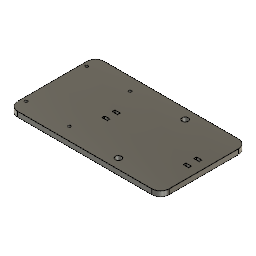
assembly v3 (Autodesk Fusion 360 archive; units mm, degrees)
design "base_assem"
Autodesk Fusion 360 part; units mm, degrees
sketch "Sketch1" plane through (0, 0, 0) normal (0, 0, 1) x (1, 0, 0)
  line L0 (10, 0) -> (165, 0)
  line L1 (175, 10) -> (175, 90)
  line L2 (165, 100) -> (10, 100)
  line L3 (0, 90) -> (0, 10)
  line L4 (5, 85) -> (55, 85)
  line L5 (55, 85) -> (55, 15)
  line L6 (55, 15) -> (5, 15)
  line L7 (5, 15) -> (5, 85)
  line L8 (5, 50) -> (0, 50)
  circle A0 centre (5, 85) radius 1.5
  circle A1 centre (55, 85) radius 1.5
  circle A2 centre (5, 15) radius 1.5
  circle A3 centre (55, 15) radius 1.5
  line L9 (55, 100) -> (55, 0)
  line L10 (65, 100) -> (65, 0)
  line L11 (165, 0) -> (165, 100)
  line L12 (65, 57.5) -> (71, 57.5)
  line L13 (71, 57.5) -> (71, 42.5)
  line L14 (71, 42.5) -> (65, 42.5)
  line L15 (65, 42.5) -> (65, 57.5)
  line L16 (65, 57.5) -> (71, 57.5)
  line L17 (71, 57.5) -> (71, 54.5)
  line L18 (71, 54.5) -> (65, 54.5)
  line L19 (65, 54.5) -> (65, 57.5)
  line L20 (71, 42.5) -> (65, 42.5)
  line L21 (65, 42.5) -> (65, 45.5)
  line L22 (65, 45.5) -> (71, 45.5)
  line L23 (71, 45.5) -> (71, 42.5)
  line L24 (65, 100) -> (165, 100)
  line L25 (115, 100) -> (115, 0)
  line L26 (159, 57.5) -> (159, 42.5)
  line L27 (159, 54.5) -> (165, 54.5)
  line L28 (165, 57.5) -> (159, 57.5)
  line L29 (165, 45.5) -> (159, 45.5)
  line L30 (159, 42.5) -> (165, 42.5)
  circle A4 centre (115, 88.5) radius 3.5
  circle A5 centre (115, 11.5) radius 3.5
  line L31 (115, 88.5) -> (115, 11.5)
  arc A6 (10, 100) -> (0, 90) centre (10, 90) ccw
  arc A7 (0, 10) -> (10, 0) centre (10, 10) ccw
  arc A8 (175, 90) -> (165, 100) centre (165, 90) ccw
  arc A9 (165, 0) -> (175, 10) centre (165, 10) ccw
  point P0 (0, 100)
  point P1 (65, 50)
  point P2 (65, 50)
  point P3 (115, 50)
  point P4 (115, 50)
  dimension "d1" = 50
  dimension "d2" = 70
  dimension "d3" = 100
  dimension "d4" = 90
  dimension "d5" = 5
  dimension "d6" = 3
  dimension "d7" = 3
  dimension "d8" = 3
  dimension "d9" = 3
  dimension "d11" = 120
  dimension "d12" = 10
  dimension "d13" = 10
  dimension "d14" = 6
  dimension "d15" = 15
  dimension "d16" = 3
  dimension "d17" = 3
  dimension "d18" = 77
  dimension "d19" = 7
  dimension "d20" = 7
  dimension "d21" = 10
  dimension "d22" = 10
  dimension "d23" = 10
  dimension "d24" = 10
  constraint horizontal L0
  constraint vertical L1
  constraint horizontal L2
  constraint vertical L3
  constraint horizontal L4
  constraint vertical L5
  constraint horizontal L6
  constraint vertical L7
  constraint midpoint L7 L8.start
  constraint coincident L4.start L7.end
  constraint coincident L4.end L5.start
  constraint coincident L6.end L7.start
  constraint coincident L5.end L6.start
  constraint coincident L0 L9.end
  constraint perpendicular L0 L9
  constraint coincident L2 L10.start
  constraint coincident L0 L10.end
  constraint perpendicular L0 L10
  constraint coincident L0 L11.start
  constraint coincident L2 L11.end
  constraint perpendicular L2 L11
  constraint coincident L4.end L9
  constraint horizontal L12
  constraint vertical L13
  constraint horizontal L14
  constraint vertical L15
  constraint horizontal L16
  constraint vertical L17
  constraint horizontal L18
  constraint vertical L19
  constraint coincident L13 L17.end
  constraint horizontal L20
  constraint vertical L21
  constraint horizontal L22
  constraint vertical L23
  constraint coincident L15 L21.end
  constraint midpoint L10 P2
  constraint midpoint L15 P2
  constraint coincident P2 P1
  constraint midpoint L24 L25.start
  constraint coincident L0 L25.end
  constraint perpendicular L0 L25
  constraint symmetric L12.start L25 L28.start
  constraint symmetric L12.end L25 L26.start
  constraint symmetric L13.end L25 L26.end
  constraint symmetric L17.end L25 L27.start
  constraint symmetric L18.end L25 L27.end
  constraint symmetric L14.end L25 L30.end
  constraint symmetric L21.end L25 L29.start
  constraint symmetric L22.end L25 L29.end
  constraint coincident L25 A4.centre
  constraint coincident L25 A5.centre
  constraint coincident A4.centre L31.start
  constraint coincident A5.centre L31.end
  constraint midpoint L31 P4
  constraint midpoint L25 P4
  constraint coincident P4 P3
  constraint coincident L3 L8.end
  constraint coincident P0 L2
  constraint coincident P0 L3
  constraint tangent L2 A6
  constraint tangent L3 A6
  constraint coincident origin L0
  constraint coincident origin L3
  constraint tangent L0 A7
  constraint tangent L3 A7
  constraint tangent L1 A8
  constraint tangent L2 A8
  constraint tangent L0 A9
  constraint tangent L1 A9
  measures "d1" distance of L4.start L4.end
  measures "d2" distance of L4.start L6.end
  measures "d3" distance of origin P0
  measures "d4" angle of L3 L8
  measures "d5" distance of L8.start L8.end
  measures "d6" diameter of A0
  measures "d7" diameter of A1
  measures "d8" diameter of A3
  measures "d9" diameter of A2
  measures "d11" distance of L1 L9
  measures "d12" distance of L9 L10
  measures "d13" distance of L1 L11
  measures "d14" distance of L12.start L12.end
  measures "d15" distance of L12.end L13.end
  measures "d16" distance of L16 L18
  measures "d17" distance of L14 L22
  measures "d18" distance of A4.centre A5.centre
  measures "d19" diameter of A4
  measures "d20" diameter of A5
  measures "d21" radius of A6
  measures "d22" radius of A7
  measures "d23" radius of A8
  measures "d24" radius of A9
extrude "Extrude1" add sketch "Sketch1" along normal blind 6 contours L0 L3 L6 L7 L8 A2 A3 L9 A7 | L0 L2 L5 A1 A3 L9 L10 L15 L19 L21 | L0 L2 L10 L12 L13 L14 L16 L17 L20 L23 L24 L25 A4 A5 L31 | L2 L3 L4 L7 L8 A0 A1 L9 A6 | L0 L2 L11 L24 L25 L26 L28 L30 A4 A5 L31 | L4 L5 L6 L7 A0 A1 A2 A3 L9 | L1 L11 A8 A9 | L10 L13 L15 L18 L22 | L11 L26 L27 L29
equation "d18 = ( ( 70 + 84 ) / 2 ) * 1 mm"

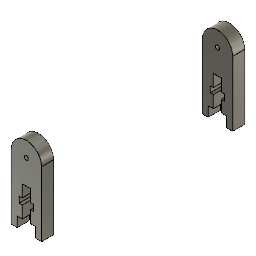
design "rotor_mount_assem"
Autodesk Fusion 360 part; units mm, degrees
sketch "Sketch1" plane through (0, 0, 0) normal (0, 1, 0) x (1, 0, 0)
  circle A0 centre (0, 0) radius 28.5
  line L0 (-9, 27.0416) -> (9, 27.0416)
  line L1 (-27.3663, -7.9584) -> (-39.2742, -7.9584)
  line L2 (-49.2742, 2.0416) -> (-49.2742, 27.0416)
  line L3 (-49.2742, 27.0416) -> (-9, 27.0416)
  line L4 (-41.2742, 27.0416) -> (-34.2742, 27.0416)
  line L5 (-34.2742, 27.0416) -> (-34.2742, 2.0416)
  line L6 (-34.2742, 2.0416) -> (-41.2742, 2.0416)
  line L7 (-41.2742, 2.0416) -> (-41.2742, 27.0416)
  line L8 (-41.2742, 2.0416) -> (-49.2742, 2.0416)
  line L9 (-49.2742, 2.0416) -> (-34.2742, 2.0416)
  line L10 (-28.4268, 2.0416) -> (-34.2742, 2.0416)
  line L11 (-44.2742, 11.0416) -> (-31.2742, 11.0416)
  line L12 (-31.2742, 11.0416) -> (-31.2742, 18.0416)
  line L13 (-31.2742, 18.0416) -> (-44.2742, 18.0416)
  line L14 (-44.2742, 18.0416) -> (-44.2742, 11.0416)
  line L15 (-37.7742, 18.0416) -> (-37.7742, 27.0416)
  line L16 (-44.2742, 14.5416) -> (-41.2742, 14.5416)
  line L17 (-44.2742, 11.0416) -> (-49.2742, 11.0416)
  line L18 (-31.2742, 11.0416) -> (-26.2742, 11.0416)
  arc A1 (-49.2742, 2.0416) -> (-39.2742, -7.9584) centre (-39.2742, 2.0416) ccw
  line L19 (0, 27.0416) -> (0, 0)
  line L20 (27.3663, -7.9584) -> (39.2742, -7.9584)
  arc A2 (39.2742, -7.9584) -> (49.2742, 2.0416) centre (39.2742, 2.0416) ccw
  line L21 (49.2742, 2.0416) -> (49.2742, 27.0416)
  line L22 (49.2742, 27.0416) -> (9, 27.0416)
  line L23 (31.2742, 18.0416) -> (44.2742, 18.0416)
  line L24 (31.2742, 11.0416) -> (31.2742, 18.0416)
  line L25 (44.2742, 11.0416) -> (31.2742, 11.0416)
  line L26 (44.2742, 18.0416) -> (44.2742, 11.0416)
  line L27 (41.2742, 2.0416) -> (41.2742, 27.0416)
  line L28 (34.2742, 27.0416) -> (34.2742, 2.0416)
  line L29 (34.2742, 2.0416) -> (41.2742, 2.0416)
  circle A3 centre (0, 0) radius 1
  circle A4 centre (0, 0) radius 7.5
  line L30 (0, 0) -> (-7.5, 0)
  line L31 (-7.5, 0) -> (-7.5, 27.0416)
  line L32 (0, 0) -> (7.5, 0)
  line L33 (7.5, 0) -> (7.5, 27.0416)
  line L34 (-2, 27.0416) -> (2, 27.0416)
  line L35 (2, 27.0416) -> (2, 12.0416)
  line L36 (2, 12.0416) -> (-2, 12.0416)
  line L37 (-2, 12.0416) -> (-2, 27.0416)
  line L38 (-3.5, 18.0416) -> (3.5, 18.0416)
  line L39 (3.5, 18.0416) -> (3.5, 21.0416)
  line L40 (3.5, 21.0416) -> (-3.5, 21.0416)
  line L41 (-3.5, 21.0416) -> (-3.5, 18.0416)
  line L42 (-2, 19.5416) -> (-3.5, 19.5416)
  line L43 (-7.5, 27.0416) -> (-4.5, 27.0416)
  line L44 (-4.5, 27.0416) -> (-4.5, 32.0416)
  line L45 (-4.5, 32.0416) -> (-7.5, 32.0416)
  line L46 (-7.5, 32.0416) -> (-7.5, 27.0416)
  line L47 (7.5, 27.0416) -> (4.5, 27.0416)
  line L48 (4.5, 27.0416) -> (4.5, 32.0416)
  line L49 (4.5, 32.0416) -> (7.5, 32.0416)
  line L50 (7.5, 32.0416) -> (7.5, 27.0416)
  point P0 (0, 21.0416)
  point P1 (0, 27.0416)
  dimension "d1" = 57
  dimension "d2" = 18
  dimension "d3" = 25
  dimension "d4" = 90
  dimension "d5" = 10
  dimension "d8" = 7
  dimension "d9" = 7
  dimension "d10" = 13
  dimension "d11" = 90
  dimension "d12" = 90
  dimension "d13" = 5
  dimension "d14" = 5
  dimension "d15" = 10
  dimension "d18" = 2
  dimension "d19" = 15
  dimension "d20" = 4
  dimension "d21" = 15
  dimension "d22" = 3
  dimension "d23" = 7
  dimension "d24" = 90
  dimension "d25" = 5
  dimension "d26" = 5
  dimension "d27" = 3
  dimension "d28" = 3
  constraint coincident A0.centre L19.end
  constraint coincident A0 L0.start
  constraint coincident A0 L0.end
  constraint horizontal L0
  constraint coincident A0 L1.start
  constraint perpendicular L0 L2
  constraint perpendicular L2 L3
  constraint horizontal L4
  constraint vertical L5
  constraint horizontal L6
  constraint vertical L7
  constraint coincident L3 L4.start
  constraint coincident L2 L8.end
  constraint perpendicular L2 L8
  constraint perpendicular L5 L9
  constraint coincident A0 L10.start
  constraint perpendicular L5 L10
  constraint horizontal L11
  constraint vertical L12
  constraint horizontal L13
  constraint vertical L14
  constraint midpoint L13 L15.start
  constraint midpoint L4 L15.end
  constraint midpoint L14 L16.start
  constraint midpoint L7 L16.end
  constraint perpendicular L2 L17
  constraint coincident A0 L18.end
  constraint perpendicular L12 L18
  constraint coincident L2 L17.end
  constraint tangent L1 A1
  constraint tangent L2 A1
  constraint midpoint L0 P1
  constraint symmetric L0.start L19 L0.end
  constraint symmetric L1.start L19 L20.start
  constraint symmetric L2.end L19 L21.end
  constraint symmetric L4.start L19 L27.end
  constraint symmetric L4.end L19 L28.start
  constraint symmetric L5.end L19 L28.end
  constraint symmetric L6.end L19 L27.start
  constraint symmetric L11.start L19 L25.start
  constraint symmetric L11.end L19 L24.start
  constraint symmetric L12.end L19 L23.start
  constraint symmetric L13.end L19 L23.end
  constraint symmetric L1.end L19 L20.end
  constraint symmetric L2.start L19 A2.end
  constraint symmetric A1 L19 A2
  constraint concentric A3 A4
  constraint coincident A4 L30.end
  constraint perpendicular L19 L30
  constraint coincident L0 L31.end
  constraint tangent A4 L31
  constraint coincident A4 L32.end
  constraint perpendicular L19 L32
  constraint coincident L0 L33.end
  constraint tangent A4 L33
  constraint horizontal L34
  constraint vertical L35
  constraint horizontal L36
  constraint vertical L37
  constraint horizontal L38
  constraint vertical L39
  constraint horizontal L40
  constraint vertical L41
  constraint midpoint L37 L42.start
  constraint midpoint L41 L42.end
  constraint midpoint L40 P0
  constraint midpoint L34 P1
  constraint coincident L19 P0
  constraint coincident P1 L19.start
  constraint horizontal L43
  constraint vertical L44
  constraint horizontal L45
  constraint vertical L46
  constraint horizontal L47
  constraint vertical L48
  constraint horizontal L49
  constraint vertical L50
  measures "d1" diameter of A0
  measures "d2" distance of L0.start L0.end
  measures "d3" distance of L4.end L5.end
  measures "d4" angle of L1 L2
  measures "d5" distance of L1 L6
  measures "d8" distance of L5 L7
  measures "d9" distance of L11.start L13.end
  measures "d10" distance of L12 L14
  measures "d11" angle of L7 L16
  measures "d12" angle of L4 L15
  measures "d13" distance of L11.end L18.end
  measures "d14" distance of L11.start L17.end
  measures "d15" radius of A1
  measures "d18" diameter of A3
  measures "d19" diameter of A4
  measures "d20" distance of L35.end L36.end
  measures "d21" distance of L34.end L35.end
  measures "d22" distance of L38.start L40.end
  measures "d23" distance of L38.start L38.end
  measures "d24" angle of L37 L42
  measures "d25" distance of L31.end L45.end
  measures "d26" distance of L33.end L49.end
  measures "d27" distance of L48.end L49.end
  measures "d28" distance of L44.end L45.end
extrude "Extrude1" add sketch "Sketch1" along normal blind 100 contours A0 L0 L47 L48 L50 | A0 L48 L49 L50 | L0 L19 A4 L33 L35 L36 L38 L39 L40 L47 | L19 A3 A4 L32 | A3 A4 L30 L32 | A0 L0 L43 L44 L46 | A0 L44 L45 L46 | L0 L19 A4 L31 L36 L37 L38 L40 L41 L43 | L19 A3 A4 L30 makes body 1
sketch "Sketch2" plane through (7.5, 0, 0) normal (1, 0, 0) x (0, 1, 0)
  line L0 (0, 0) -> (0, -32.0416)
  line L1 (0, -32.0416) -> (100, -32.0416)
  line L2 (100, -32.0416) -> (100, 0)
  line L3 (100, 0) -> (0, 0)
  line L4 (5, 18.4454) -> (95, 18.4454)
  line L5 (95, 18.4454) -> (95, -40)
  line L6 (95, -40) -> (5, -40)
  line L7 (5, -40) -> (5, 18.4454)
  dimension "d29" = 5
  dimension "d30" = 5
  constraint horizontal L4
  constraint vertical L5
  constraint horizontal L6
  constraint vertical L7
  measures "d29" distance of L0 L7
  measures "d30" distance of L2 L5
extrude "Extrude2" cut sketch "Sketch2" against normal blind 100 contours L3 L4 L5 L7 | L1 L3 L5 L7 bodies 1 makes body 2 at (-3.3745, 100, -4.2745)
extrude "Extrude3" add 1 faces at (-3.3745, 5, -4.2745) along direction (0, 1, 0) blind 1 on bodies 1 bodies 1
extrude "Extrude4" add 1 faces at (-3.3745, 95, -4.2745) along direction (0, -1, 0) blind 1 on bodies 2 bodies 2

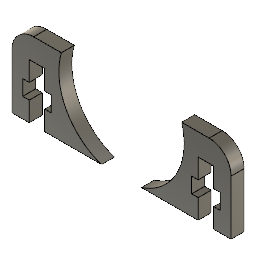
design "stator_mount_assem"
Autodesk Fusion 360 part; units mm, degrees
sketch "Sketch1" plane through (0, 0, 0) normal (0, 1, 0) x (1, 0, 0)
  circle A0 centre (0, 0) radius 28.5
  line L0 (-9, 27.0416) -> (9, 27.0416)
  line L1 (-27.3663, -7.9584) -> (-40, -7.9584)
  line L2 (-50, 2.0416) -> (-50, 27.0416)
  line L3 (-50, 27.0416) -> (-9, 27.0416)
  line L4 (-42, 27.0416) -> (-35, 27.0416)
  line L5 (-35, 27.0416) -> (-35, 2.0416)
  line L6 (-35, 2.0416) -> (-42, 2.0416)
  line L7 (-42, 2.0416) -> (-42, 27.0416)
  line L8 (-42, 2.0416) -> (-50, 2.0416)
  line L9 (-50, 2.0416) -> (-35, 2.0416)
  line L10 (-28.4268, 2.0416) -> (-35, 2.0416)
  line L11 (-45, 11.0416) -> (-32, 11.0416)
  line L12 (-32, 11.0416) -> (-32, 18.0416)
  line L13 (-32, 18.0416) -> (-45, 18.0416)
  line L14 (-45, 18.0416) -> (-45, 11.0416)
  line L15 (-38.5, 18.0416) -> (-38.5, 27.0416)
  line L16 (-45, 14.5416) -> (-42, 14.5416)
  line L17 (-45, 11.0416) -> (-50, 11.0416)
  line L18 (-32, 11.0416) -> (-26.2742, 11.0416)
  arc A1 (-50, 2.0416) -> (-40, -7.9584) centre (-40, 2.0416) ccw
  line L19 (0, 27.0416) -> (0, 0)
  line L20 (27.3663, -7.9584) -> (40, -7.9584)
  arc A2 (40, -7.9584) -> (50, 2.0416) centre (40, 2.0416) ccw
  line L21 (50, 2.0416) -> (50, 27.0416)
  line L22 (50, 27.0416) -> (9, 27.0416)
  line L23 (32, 18.0416) -> (45, 18.0416)
  line L24 (32, 11.0416) -> (32, 18.0416)
  line L25 (45, 11.0416) -> (32, 11.0416)
  line L26 (45, 18.0416) -> (45, 11.0416)
  line L27 (42, 2.0416) -> (42, 27.0416)
  line L28 (35, 27.0416) -> (35, 2.0416)
  line L29 (35, 2.0416) -> (42, 2.0416)
  dimension "d1" = 57
  dimension "d2" = 18
  dimension "d3" = 25
  dimension "d4" = 90
  dimension "d5" = 10
  dimension "d8" = 7
  dimension "d9" = 7
  dimension "d10" = 13
  dimension "d11" = 90
  dimension "d12" = 90
  dimension "d15" = 10
  dimension "d18" = 100
  dimension "d20" = 5
  constraint coincident A0.centre L19.end
  constraint coincident A0 L0.start
  constraint coincident A0 L0.end
  constraint horizontal L0
  constraint coincident A0 L1.start
  constraint perpendicular L0 L2
  constraint perpendicular L2 L3
  constraint horizontal L4
  constraint vertical L5
  constraint horizontal L6
  constraint vertical L7
  constraint coincident L3 L4.start
  constraint coincident L2 L8.end
  constraint perpendicular L2 L8
  constraint perpendicular L5 L9
  constraint coincident A0 L10.start
  constraint perpendicular L5 L10
  constraint horizontal L11
  constraint vertical L12
  constraint horizontal L13
  constraint vertical L14
  constraint midpoint L13 L15.start
  constraint midpoint L4 L15.end
  constraint midpoint L14 L16.start
  constraint midpoint L7 L16.end
  constraint perpendicular L2 L17
  constraint coincident A0 L18.end
  constraint perpendicular L12 L18
  constraint coincident L2 L17.end
  constraint tangent L1 A1
  constraint tangent L2 A1
  constraint midpoint L0 L19.start
  constraint symmetric L0.start L19 L0.end
  constraint symmetric L1.start L19 L20.start
  constraint symmetric L2.end L19 L21.end
  constraint symmetric L4.start L19 L27.end
  constraint symmetric L4.end L19 L28.start
  constraint symmetric L5.end L19 L28.end
  constraint symmetric L6.end L19 L27.start
  constraint symmetric L11.start L19 L25.start
  constraint symmetric L11.end L19 L24.start
  constraint symmetric L12.end L19 L23.start
  constraint symmetric L13.end L19 L23.end
  constraint symmetric L1.end L19 L20.end
  constraint symmetric L2.start L19 A2.end
  constraint symmetric A1 L19 A2
  measures "d1" diameter of A0
  measures "d2" distance of L0.start L0.end
  measures "d3" distance of L4.end L5.end
  measures "d4" angle of L1 L2
  measures "d5" distance of L1 L6
  measures "d8" distance of L5 L7
  measures "d9" distance of L11.start L13.end
  measures "d10" distance of L12 L14
  measures "d11" angle of L7 L16
  measures "d12" angle of L4 L15
  measures "d15" radius of A1
  measures "d18" distance of L2 L21
  measures "d20" distance of L11.start L17.end
extrude "Extrude1" add sketch "Sketch1" along normal blind 5 contours A0 L20 A2 L21 L22 L23 L24 L25 L26 L27 L28 L29 | A0 L3 L5 L12 L13 L18 | A0 L1 L6 L8 L9 L10 A1 | A0 L5 L10 L11 L18 | L2 L7 L8 L9 L11 L17 | L2 L3 L7 L13 L14 L17 makes body 1 at (-34.4021, 5, 3.3326) makes body 2 at (34.4021, 5, 3.3326)
extrude "Extrude2" add 2 faces at (-34.4021, 0, 3.3326) (34.4021, 0, 3.3326) along direction (0, -1, 0) blind 1 on bodies 1 2 bodies 1 2

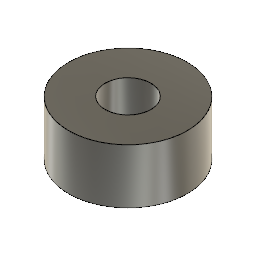
design "washer"
Autodesk Fusion 360 part; units mm, degrees
sketch "Sketch1" plane through (0, 0, 0) normal (0, 0, 1) x (1, 0, 0)
  circle A0 centre (0, 0) radius 1.25
  circle A1 centre (0, 0) radius 3.25
  dimension "d1" = 2.5
  dimension "d2" = 2
  constraint coincident A0.centre A1.centre
  constraint concentric A0 A1
  measures "d1" diameter of A0
  measures "d2" distance of A0 A1
extrude "Extrude1" add sketch "Sketch1" along normal blind 3
